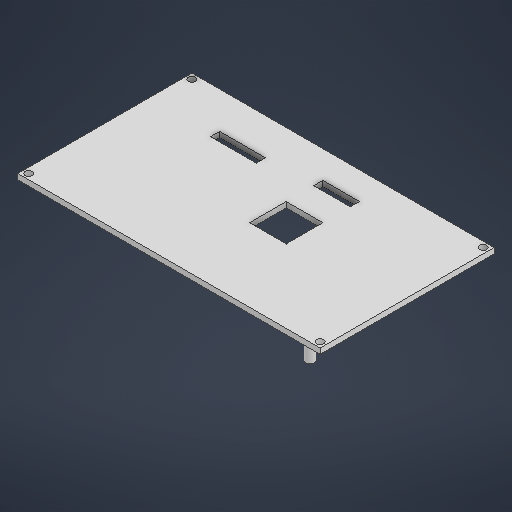
# Autodesk Inventor part: 零件2
Saved by Autodesk Inventor 2026.2 (Build 302298000, 298)
## iProperties
Created: 2025-12-21
Part Number: 零件2
Material: 一般
Document SubType Name: Modeling
Designer: USER
Density: 1 g/cm^3
Appearance: 預設
Author: USER
Autodesk Inventor part; units mm, degrees
ref_plane "YZ Plane" through (0, 0, 0) normal (1, 0, 0) x (0, 1, 0)
ref_plane "XZ Plane" through (0, 0, 0) normal (0, 1, 0) x (-1, 0, 0)
ref_plane "XY Plane" through (0, 0, 0) normal (0, 0, 1) x (1, 0, 0)
sketch "草圖1" plane through (0, 0, 0) normal (0, 1, 0) x (-1, 0, 0)
  line L0 (0, 0) -> (-165, 0)
  line L1 (-165, 0) -> (-165, -95)
  line L2 (-165, -95) -> (0, -95)
  line L3 (0, -95) -> (0, 0)
  dimension "d0" = 165
  dimension "d1" = 95
  constraints: 8 end point, 2 parallel, 1 horizontal, 1 perpendicular
  measures "d0" distance of L1.end L2.end
  measures "d1" distance of L0.end L1.end
extrude "擠出1" add sketch "草圖1" along normal blind 3
sketch "草圖2" plane through (0, 3, 0) normal (0, 1, 0) x (1, 0, 0)
  line L0 (30, 75) -> (65, 75)
  line L1 (65, 75) -> (65, 20)
  line L2 (65, 20) -> (30, 20)
  line L3 (30, 20) -> (30, 75)
  line L4 (0, 95) -> (0, 0) projected
  line L5 (165, 95) -> (0, 95) projected
  line L6 (35.1505, 75) -> (60.1505, 75)
  line L7 (60.1505, 75) -> (60.1505, 70)
  line L8 (60.1505, 70) -> (35.1505, 70)
  line L9 (35.1505, 70) -> (35.1505, 75)
  dimension "d4" = 55
  dimension "d5" = 35
  dimension "d6" = 30
  dimension "d7" = 20
  dimension "d8" = 25
  dimension "d9" = 5
  dimension "d10" = 0
  constraints: 16 end point, 4 parallel, 2 horizontal, 2 perpendicular
  measures "d4" distance of L2.end L0.start
  measures "d5" distance of L0.start L0.end
  measures "d6" distance between parallel lines of L4 L3
  measures "d7" distance between parallel lines of L5 L0
  measures "d8" distance of L6.start L6.end
  measures "d9" distance of L6.end L7.end
  measures "d10" distance between parallel lines of L0 L6
extrude "擠出2" cut sketch "草圖2" against normal blind 3 contours L0 L7 L8 L9
sketch "草圖3" plane through (0, 3, 0) normal (0, 1, 0) x (1, 0, 0)
  line L0 (86.5, 60) -> (106.5, 60)
  line L1 (106.5, 60) -> (106.5, 40)
  line L2 (106.5, 40) -> (86.5, 40)
  line L3 (86.5, 40) -> (86.5, 60)
  line L4 (85, 55) -> (108, 55)
  line L5 (108, 55) -> (108, 10)
  line L6 (108, 10) -> (85, 10)
  line L7 (85, 10) -> (85, 55)
  line L8 (165, 0) -> (165, 95) projected
  line L9 (0, 0) -> (165, 0) projected
  dimension "d13" = 20
  dimension "d14" = 20
  dimension "d15" = 23
  dimension "d16" = 45
  dimension "d17" = 80
  dimension "d18" = 1.5
  dimension "d19" = 30
  dimension "d20" = 10
  constraints: 16 end point, 4 parallel, 2 horizontal, 2 perpendicular
  measures "d13" distance of L2.end L0.start
  measures "d14" distance of L0.start L0.end
  measures "d15" distance of L5.end L6.end
  measures "d16" distance of L4.end L5.end
  measures "d17" distance between parallel lines of L8 L7
  measures "d18" distance between parallel lines of L7 L3
  measures "d19" distance between parallel lines of L6 L2
  measures "d20" distance between parallel lines of L9 L6
extrude "擠出3" cut sketch "草圖3" against normal blind 3 contours L0 L1 L4 L3 | L4 L1 L2 L3
sketch "草圖4" plane through (0, 3, 0) normal (0, 1, 0) x (1, 0, 0)
  line L0 (86.5, 80) -> (106.5, 80)
  line L1 (106.5, 80) -> (106.5, 75)
  line L2 (106.5, 75) -> (86.5, 75)
  line L3 (86.5, 75) -> (86.5, 80)
  line L4 (86.5, 40) -> (86.5, 60) projected
  line L5 (106.5, 60) -> (106.5, 40) projected
  line L6 (86.5, 60) -> (106.5, 60) projected
  point P0 (0, 0)
  dimension "d23" = 0
  dimension "d24" = 0
  dimension "d25" = 5
  dimension "d26" = 15
  constraints: 8 end point, 2 parallel, 1 horizontal, 1 perpendicular
  measures "d23" distance between parallel lines of L4 L3
  measures "d24" distance between parallel lines of L5 L1
  measures "d25" distance of L0.end L1.end
  measures "d26" distance between parallel lines of L6 L2
extrude "擠出4" cut sketch "草圖4" against normal blind 3
sketch "草圖5" plane through (0, 3, 0) normal (0, 1, 0) x (1, 0, 0)
  circle A0 centre (3, 3) radius 2
  line L0 (0, 95) -> (0, 0) projected
  line L1 (0, 0) -> (165, 0) projected
  circle A1 centre (3, 92) radius 2
  line L2 (165, 95) -> (0, 95) projected
  circle A2 centre (162, 92) radius 2
  line L3 (165, 0) -> (165, 95) projected
  circle A3 centre (162, 3) radius 2
  dimension "d29" = 4
  dimension "d30" = 3
  dimension "d31" = 3
  dimension "d32" = 4
  dimension "d33" = 3
  dimension "d34" = 3
  dimension "d35" = 4
  dimension "d36" = 3
  dimension "d37" = 3
  dimension "d38" = 4
  dimension "d39" = 3
  dimension "d40" = 3
  constraints: 4 centre point
  measures "d29" diameter of A0
  measures "d30" distance from line of L0 A0.centre
  measures "d31" distance from line of L1 A0.centre
  measures "d32" diameter of A1
  measures "d33" distance from line of L2 A1.centre
  measures "d34" distance from line of L0 A1.centre
  measures "d35" diameter of A2
  measures "d36" distance from line of L2 A2.centre
  measures "d37" distance from line of L3 A2.centre
  measures "d38" diameter of A3
  measures "d39" distance from line of L3 A3.centre
  measures "d40" distance from line of L1 A3.centre
extrude "擠出5" cut sketch "草圖5" against normal blind 5 contours A0 | A1 | A2 | A3
sketch "草圖6" plane through (0, 0, 0) normal (0, -1, 0) x (1, 0, 0)
  circle A0 centre (125, -34.5) radius 2.5
  line L0 (165, 0) -> (165, -95) projected
  line L1 (0, 0) -> (165, 0) projected
  dimension "d43" = 5
  dimension "d44" = 40
  dimension "d45" = 32
  constraints: 1 centre point
  measures "d43" diameter of A0
  measures "d44" distance from line of A0.centre L0
  measures "d45" distance edge to line of A0 L1
extrude "擠出6" add sketch "草圖6" along normal blind 40
